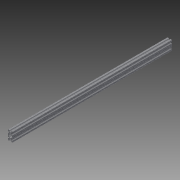
# Autodesk Inventor part: 1530-50_5
Saved by Autodesk Inventor 2013 (Build 170138000, 138)
## iProperties
Category: PARTsolutions
Company: 8020
Created: 2013-09-15
Part Number: 1530-50_5
Catalog Web Link: www.cadenas.de
Description: 1530-T-Slotted Profile - 15 Series
Vendor: 8020
Document SubType Name: Modeling
Designer: PARTuser1
Manufacturer: 8020
Density: 1 g/cm^3
Material: Generic
Mass: 1722.42 g
Surface Area: 7668.33 cm^2
Volume: 1722.42 cm^3
PSOL_IDENT_0: {$CADENAS_DATA\23d-libs\8020\inch\profiles\15_series\1530.prj},149 {VTYP=3D},{NB=1530-97},{LINA=1530
PSOL_IDENT_1: -97},{NN=1530},{DATE=22.08.2012},{GEOMDATE=16.08.2012 10:03:00},{VERSION=},{LINEID=10},{LINESUBID=-1
PSOL_IDENT_2: },{WBVAR=LS,L}  {NB=1530-97},{LINA=1530-97},{KT=DUMMY},{PN=1530-97},{SERIES=1530},{MAT=6105-T5 Alumi
PSOL_IDENT_3: num},{FIN=Clear Anodize},{LS=},{L=97.000},{LALG=97,145,242},{W=2.4209},{MIX=1.8042},{MIY=.4824},{EA=
PSOL_IDENT_4: 2.0798}
CNS_NT: T-Slotted Profile - 15 Series
CNS_NB: 1530-97
CNS_NBSYN: $PN.$LS.
CNS_LINA: 1530-97
CNS_PN: 1530-97
CNS_SERIES: 1530
CNS_MAT: 6105-T5 Aluminum
CNS_FIN: Clear Anodize
CNS_LS: Stock Length
CNS_L: 97.000
CNS_LALG: 97,145,242
CNS_W: 2.4209
CNS_MIX: 1.8042
CNS_MIY: .4824
CNS_EA: 2.0798
SUPPLIER: 8020
ARTICLENO: 1530-97
BOMINFO: 1530-97
CREATOR: CADENAS GmbH
Title: 1530-97
Author: Cadenas PARTsolutions
Comments: T-Slotted Profile - 15 Series
Autodesk Inventor part; units mm, degrees
sketch "Sketch_1" plane through (0, 0, 0) normal (0, 0, 1) x (1, 0, 0)
  arc A0 (-19.05, -15.8496) -> (-19.05, -14.3256) centre (-19.05, -15.0876) ccw
  line L0 (-19.05, -15.8496) -> (-19.05, -15.875)
  arc A1 (-19.05, -15.875) -> (-15.875, -19.05) centre (-15.875, -15.875) ccw
  line L1 (-15.875, -19.05) -> (-15.8496, -19.05)
  arc A2 (-14.3256, -19.05) -> (-15.8496, -19.05) centre (-15.0876, -19.05) ccw
  line L2 (-14.3256, -19.05) -> (-9.4996, -19.05)
  arc A3 (-7.9756, -19.05) -> (-9.4996, -19.05) centre (-8.7376, -19.05) ccw
  line L3 (-7.9756, -19.05) -> (-5.6388, -19.05)
  arc A4 (-5.6388, -19.05) -> (-4.064, -17.4752) centre (-5.6388, -17.4752) ccw
  line L4 (-4.064, -17.4752) -> (-4.064, -16.5608)
  arc A5 (-4.064, -16.5608) -> (-5.6388, -14.986) centre (-5.6388, -16.5608) ccw
  line L5 (-5.6388, -14.986) -> (-9.398, -14.986)
  arc A6 (-10.287, -14.097) -> (-9.398, -14.986) centre (-9.398, -14.097) ccw
  line L6 (-10.287, -14.097) -> (-10.287, -13.5289)
  arc A7 (-10.0266, -12.9003) -> (-10.287, -13.5289) centre (-9.398, -13.5289) ccw
  line L7 (-10.0266, -12.9003) -> (-5.2739, -8.1476)
  arc A8 (-1.9153, -6.7564) -> (-5.2739, -8.1476) centre (-1.9153, -11.5062) ccw
  line L8 (-1.9153, -6.7564) -> (1.9153, -6.7564)
  arc A9 (5.2739, -8.1476) -> (1.9153, -6.7564) centre (1.9153, -11.5062) ccw
  line L9 (5.2739, -8.1476) -> (10.0266, -12.9003)
  arc A10 (10.287, -13.5289) -> (10.0266, -12.9003) centre (9.398, -13.5289) ccw
  line L10 (10.287, -13.5289) -> (10.287, -14.097)
  arc A11 (9.398, -14.986) -> (10.287, -14.097) centre (9.398, -14.097) ccw
  line L11 (9.398, -14.986) -> (5.6388, -14.986)
  arc A12 (5.6388, -14.986) -> (4.064, -16.5608) centre (5.6388, -16.5608) ccw
  line L12 (4.064, -16.5608) -> (4.064, -17.4752)
  arc A13 (4.064, -17.4752) -> (5.6388, -19.05) centre (5.6388, -17.4752) ccw
  line L13 (5.6388, -19.05) -> (7.9756, -19.05)
  arc A14 (9.4996, -19.05) -> (7.9756, -19.05) centre (8.7376, -19.05) ccw
  line L14 (9.4996, -19.05) -> (12.7, -19.05)
  line L15 (12.7, -19.05) -> (14.3256, -19.05)
  arc A15 (15.8496, -19.05) -> (14.3256, -19.05) centre (15.0876, -19.05) ccw
  line L16 (15.8496, -19.05) -> (15.875, -19.05)
  arc A16 (15.875, -19.05) -> (19.05, -15.875) centre (15.875, -15.875) ccw
  line L17 (19.05, -15.875) -> (19.05, -15.8496)
  arc A17 (19.05, -14.3256) -> (19.05, -15.8496) centre (19.05, -15.0876) ccw
  line L18 (19.05, -14.3256) -> (19.05, -12.7)
  line L19 (19.05, -12.7) -> (19.05, -9.4996)
  arc A18 (19.05, -7.9756) -> (19.05, -9.4996) centre (19.05, -8.7376) ccw
  line L20 (19.05, -7.9756) -> (19.05, -5.6388)
  arc A19 (19.05, -5.6388) -> (17.4752, -4.064) centre (17.4752, -5.6388) ccw
  line L21 (17.4752, -4.064) -> (16.5608, -4.064)
  arc A20 (16.5608, -4.064) -> (14.986, -5.6388) centre (16.5608, -5.6388) ccw
  line L22 (14.986, -5.6388) -> (14.986, -9.398)
  arc A21 (14.097, -10.287) -> (14.986, -9.398) centre (14.097, -9.398) ccw
  line L23 (14.097, -10.287) -> (13.5289, -10.287)
  arc A22 (12.9003, -10.0266) -> (13.5289, -10.287) centre (13.5289, -9.398) ccw
  line L24 (12.9003, -10.0266) -> (8.1476, -5.2739)
  arc A23 (6.7564, -1.9153) -> (8.1476, -5.2739) centre (11.5062, -1.9153) ccw
  line L25 (6.7564, -1.9153) -> (6.7564, 1.9153)
  arc A24 (8.1476, 5.2739) -> (6.7564, 1.9153) centre (11.5062, 1.9153) ccw
  line L26 (8.1476, 5.2739) -> (12.9003, 10.0266)
  arc A25 (13.5289, 10.287) -> (12.9003, 10.0266) centre (13.5289, 9.398) ccw
  line L27 (13.5289, 10.287) -> (14.097, 10.287)
  arc A26 (14.986, 9.398) -> (14.097, 10.287) centre (14.097, 9.398) ccw
  line L28 (14.986, 9.398) -> (14.986, 5.6388)
  arc A27 (14.986, 5.6388) -> (16.5608, 4.064) centre (16.5608, 5.6388) ccw
  line L29 (16.5608, 4.064) -> (17.4752, 4.064)
  arc A28 (17.4752, 4.064) -> (19.05, 5.6388) centre (17.4752, 5.6388) ccw
  line L30 (19.05, 5.6388) -> (19.05, 7.9756)
  arc A29 (19.05, 9.4996) -> (19.05, 7.9756) centre (19.05, 8.7376) ccw
  line L31 (19.05, 9.4996) -> (19.05, 12.7)
  line L32 (19.05, 12.7) -> (19.05, 14.3256)
  arc A30 (19.05, 15.8496) -> (19.05, 14.3256) centre (19.05, 15.0876) ccw
  line L33 (19.05, 15.8496) -> (19.05, 22.2504)
  arc A31 (19.05, 23.7744) -> (19.05, 22.2504) centre (19.05, 23.0124) ccw
  line L34 (19.05, 23.7744) -> (19.05, 25.4)
  line L35 (19.05, 25.4) -> (19.05, 28.6004)
  arc A32 (19.05, 30.1244) -> (19.05, 28.6004) centre (19.05, 29.3624) ccw
  line L36 (19.05, 30.1244) -> (19.05, 32.4612)
  arc A33 (19.05, 32.4612) -> (17.4752, 34.036) centre (17.4752, 32.4612) ccw
  line L37 (17.4752, 34.036) -> (16.5608, 34.036)
  arc A34 (16.5608, 34.036) -> (14.986, 32.4612) centre (16.5608, 32.4612) ccw
  line L38 (14.986, 32.4612) -> (14.986, 28.702)
  arc A35 (14.097, 27.813) -> (14.986, 28.702) centre (14.097, 28.702) ccw
  line L39 (14.097, 27.813) -> (13.5289, 27.813)
  arc A36 (12.9003, 28.0734) -> (13.5289, 27.813) centre (13.5289, 28.702) ccw
  line L40 (12.9003, 28.0734) -> (8.1476, 32.8261)
  arc A37 (6.7564, 36.1847) -> (8.1476, 32.8261) centre (11.5062, 36.1847) ccw
  line L41 (6.7564, 36.1847) -> (6.7564, 40.0153)
  arc A38 (8.1476, 43.3739) -> (6.7564, 40.0153) centre (11.5062, 40.0153) ccw
  line L42 (8.1476, 43.3739) -> (12.9003, 48.1266)
  arc A39 (13.5289, 48.387) -> (12.9003, 48.1266) centre (13.5289, 47.498) ccw
  line L43 (13.5289, 48.387) -> (14.097, 48.387)
  arc A40 (14.986, 47.498) -> (14.097, 48.387) centre (14.097, 47.498) ccw
  line L44 (14.986, 47.498) -> (14.986, 43.7388)
  arc A41 (14.986, 43.7388) -> (16.5608, 42.164) centre (16.5608, 43.7388) ccw
  line L45 (16.5608, 42.164) -> (17.4752, 42.164)
  arc A42 (17.4752, 42.164) -> (19.05, 43.7388) centre (17.4752, 43.7388) ccw
  line L46 (19.05, 43.7388) -> (19.05, 46.0756)
  arc A43 (19.05, 47.5996) -> (19.05, 46.0756) centre (19.05, 46.8376) ccw
  line L47 (19.05, 47.5996) -> (19.05, 50.8)
  line L48 (19.05, 50.8) -> (19.05, 52.4256)
  arc A44 (19.05, 53.9496) -> (19.05, 52.4256) centre (19.05, 53.1876) ccw
  line L49 (19.05, 53.9496) -> (19.05, 53.975)
  arc A45 (19.05, 53.975) -> (15.875, 57.15) centre (15.875, 53.975) ccw
  line L50 (15.875, 57.15) -> (15.8496, 57.15)
  arc A46 (14.3256, 57.15) -> (15.8496, 57.15) centre (15.0876, 57.15) ccw
  line L51 (14.3256, 57.15) -> (12.7, 57.15)
  line L52 (12.7, 57.15) -> (9.4996, 57.15)
  arc A47 (7.9756, 57.15) -> (9.4996, 57.15) centre (8.7376, 57.15) ccw
  line L53 (7.9756, 57.15) -> (5.6388, 57.15)
  arc A48 (5.6388, 57.15) -> (4.064, 55.5752) centre (5.6388, 55.5752) ccw
  line L54 (4.064, 55.5752) -> (4.064, 54.6608)
  arc A49 (4.064, 54.6608) -> (5.6388, 53.086) centre (5.6388, 54.6608) ccw
  line L55 (5.6388, 53.086) -> (9.398, 53.086)
  arc A50 (10.287, 52.197) -> (9.398, 53.086) centre (9.398, 52.197) ccw
  line L56 (10.287, 52.197) -> (10.287, 51.6289)
  arc A51 (10.0266, 51.0003) -> (10.287, 51.6289) centre (9.398, 51.6289) ccw
  line L57 (10.0266, 51.0003) -> (5.2739, 46.2476)
  arc A52 (1.9153, 44.8564) -> (5.2739, 46.2476) centre (1.9153, 49.6062) ccw
  line L58 (1.9153, 44.8564) -> (-1.9153, 44.8564)
  arc A53 (-5.2739, 46.2476) -> (-1.9153, 44.8564) centre (-1.9153, 49.6062) ccw
  line L59 (-5.2739, 46.2476) -> (-10.0266, 51.0003)
  arc A54 (-10.287, 51.6289) -> (-10.0266, 51.0003) centre (-9.398, 51.6289) ccw
  line L60 (-10.287, 51.6289) -> (-10.287, 52.197)
  arc A55 (-9.398, 53.086) -> (-10.287, 52.197) centre (-9.398, 52.197) ccw
  line L61 (-9.398, 53.086) -> (-5.6388, 53.086)
  arc A56 (-5.6388, 53.086) -> (-4.064, 54.6608) centre (-5.6388, 54.6608) ccw
  line L62 (-4.064, 54.6608) -> (-4.064, 55.5752)
  arc A57 (-4.064, 55.5752) -> (-5.6388, 57.15) centre (-5.6388, 55.5752) ccw
  line L63 (-5.6388, 57.15) -> (-7.9756, 57.15)
  arc A58 (-9.4996, 57.15) -> (-7.9756, 57.15) centre (-8.7376, 57.15) ccw
  line L64 (-9.4996, 57.15) -> (-12.7, 57.15)
  line L65 (-12.7, 57.15) -> (-14.3256, 57.15)
  arc A59 (-15.8496, 57.15) -> (-14.3256, 57.15) centre (-15.0876, 57.15) ccw
  line L66 (-15.8496, 57.15) -> (-15.875, 57.15)
  arc A60 (-15.875, 57.15) -> (-19.05, 53.975) centre (-15.875, 53.975) ccw
  line L67 (-19.05, 53.975) -> (-19.05, 53.9496)
  arc A61 (-19.05, 52.4256) -> (-19.05, 53.9496) centre (-19.05, 53.1876) ccw
  line L68 (-19.05, 52.4256) -> (-19.05, 50.8)
  line L69 (-19.05, 50.8) -> (-19.05, 47.5996)
  arc A62 (-19.05, 46.0756) -> (-19.05, 47.5996) centre (-19.05, 46.8376) ccw
  line L70 (-19.05, 46.0756) -> (-19.05, 43.7388)
  arc A63 (-19.05, 43.7388) -> (-17.4752, 42.164) centre (-17.4752, 43.7388) ccw
  line L71 (-17.4752, 42.164) -> (-16.5608, 42.164)
  arc A64 (-16.5608, 42.164) -> (-14.986, 43.7388) centre (-16.5608, 43.7388) ccw
  line L72 (-14.986, 43.7388) -> (-14.986, 47.498)
  arc A65 (-14.097, 48.387) -> (-14.986, 47.498) centre (-14.097, 47.498) ccw
  line L73 (-14.097, 48.387) -> (-13.5289, 48.387)
  arc A66 (-12.9003, 48.1266) -> (-13.5289, 48.387) centre (-13.5289, 47.498) ccw
  line L74 (-12.9003, 48.1266) -> (-8.1476, 43.3739)
  arc A67 (-6.7564, 40.0153) -> (-8.1476, 43.3739) centre (-11.5062, 40.0153) ccw
  line L75 (-6.7564, 40.0153) -> (-6.7564, 36.1847)
  arc A68 (-8.1476, 32.8261) -> (-6.7564, 36.1847) centre (-11.5062, 36.1847) ccw
  line L76 (-8.1476, 32.8261) -> (-12.9003, 28.0734)
  arc A69 (-13.5289, 27.813) -> (-12.9003, 28.0734) centre (-13.5289, 28.702) ccw
  line L77 (-13.5289, 27.813) -> (-14.097, 27.813)
  arc A70 (-14.986, 28.702) -> (-14.097, 27.813) centre (-14.097, 28.702) ccw
  line L78 (-14.986, 28.702) -> (-14.986, 32.4612)
  arc A71 (-14.986, 32.4612) -> (-16.5608, 34.036) centre (-16.5608, 32.4612) ccw
  line L79 (-16.5608, 34.036) -> (-17.4752, 34.036)
  arc A72 (-17.4752, 34.036) -> (-19.05, 32.4612) centre (-17.4752, 32.4612) ccw
  line L80 (-19.05, 32.4612) -> (-19.05, 30.1244)
  arc A73 (-19.05, 28.6004) -> (-19.05, 30.1244) centre (-19.05, 29.3624) ccw
  line L81 (-19.05, 28.6004) -> (-19.05, 25.4)
  line L82 (-19.05, 25.4) -> (-19.05, 23.7744)
  arc A74 (-19.05, 22.2504) -> (-19.05, 23.7744) centre (-19.05, 23.0124) ccw
  line L83 (-19.05, 22.2504) -> (-19.05, 15.8496)
  arc A75 (-19.05, 14.3256) -> (-19.05, 15.8496) centre (-19.05, 15.0876) ccw
  line L84 (-19.05, 14.3256) -> (-19.05, 12.7)
  line L85 (-19.05, 12.7) -> (-19.05, 9.4996)
  arc A76 (-19.05, 7.9756) -> (-19.05, 9.4996) centre (-19.05, 8.7376) ccw
  line L86 (-19.05, 7.9756) -> (-19.05, 5.6388)
  arc A77 (-19.05, 5.6388) -> (-17.4752, 4.064) centre (-17.4752, 5.6388) ccw
  line L87 (-17.4752, 4.064) -> (-16.5608, 4.064)
  arc A78 (-16.5608, 4.064) -> (-14.986, 5.6388) centre (-16.5608, 5.6388) ccw
  line L88 (-14.986, 5.6388) -> (-14.986, 9.398)
  arc A79 (-14.097, 10.287) -> (-14.986, 9.398) centre (-14.097, 9.398) ccw
  line L89 (-14.097, 10.287) -> (-13.5289, 10.287)
  arc A80 (-12.9003, 10.0266) -> (-13.5289, 10.287) centre (-13.5289, 9.398) ccw
  line L90 (-12.9003, 10.0266) -> (-8.1476, 5.2739)
  arc A81 (-6.7564, 1.9153) -> (-8.1476, 5.2739) centre (-11.5062, 1.9153) ccw
  line L91 (-6.7564, 1.9153) -> (-6.7564, -1.9153)
  arc A82 (-8.1476, -5.2739) -> (-6.7564, -1.9153) centre (-11.5062, -1.9153) ccw
  line L92 (-8.1476, -5.2739) -> (-12.9003, -10.0266)
  arc A83 (-13.5289, -10.287) -> (-12.9003, -10.0266) centre (-13.5289, -9.398) ccw
  line L93 (-13.5289, -10.287) -> (-14.097, -10.287)
  arc A84 (-14.986, -9.398) -> (-14.097, -10.287) centre (-14.097, -9.398) ccw
  line L94 (-14.986, -9.398) -> (-14.986, -5.6388)
  arc A85 (-14.986, -5.6388) -> (-16.5608, -4.064) centre (-16.5608, -5.6388) ccw
  line L95 (-16.5608, -4.064) -> (-17.4752, -4.064)
  arc A86 (-17.4752, -4.064) -> (-19.05, -5.6388) centre (-17.4752, -5.6388) ccw
  line L96 (-19.05, -5.6388) -> (-19.05, -7.9756)
  arc A87 (-19.05, -9.4996) -> (-19.05, -7.9756) centre (-19.05, -8.7376) ccw
  line L97 (-19.05, -9.4996) -> (-19.05, -12.7)
  line L98 (-19.05, -12.7) -> (-19.05, -14.3256)
  circle A88 centre (0, 38.1) radius 3.3274
  circle A89 centre (0, 0) radius 3.3274
  arc A90 (-14.1109, 21.1155) -> (-14.1109, 16.9845) centre (-12.0454, 19.05) ccw
  line L99 (-14.1109, 16.9845) -> (-5.2739, 8.1476)
  arc A91 (-5.2739, 8.1476) -> (-1.9153, 6.7564) centre (-1.9153, 11.5062) ccw
  line L100 (-1.9153, 6.7564) -> (1.9153, 6.7564)
  arc A92 (1.9153, 6.7564) -> (5.2739, 8.1476) centre (1.9153, 11.5062) ccw
  line L101 (5.2739, 8.1476) -> (14.1109, 16.9845)
  arc A93 (14.1109, 16.9845) -> (14.1109, 21.1155) centre (12.0454, 19.05) ccw
  line L102 (14.1109, 21.1155) -> (5.2739, 29.9524)
  arc A94 (5.2739, 29.9524) -> (1.9153, 31.3436) centre (1.9153, 26.5938) ccw
  line L103 (1.9153, 31.3436) -> (-1.9153, 31.3436)
  arc A95 (-1.9153, 31.3436) -> (-5.2739, 29.9524) centre (-1.9153, 26.5938) ccw
  line L104 (-5.2739, 29.9524) -> (-14.1109, 21.1155)
  constraints: 210 end point, 188 point on circle, 96 centre point
extrude "Extrusion1" add sketch "Sketch_1" against normal blind 1282.7
ref_plane "b1_XY" through (0, -19.05, -1231.9) normal (0, 1, 0) x (1, 0, 0)
ref_plane "b1_YZ" through (0, -19.05, -1231.9) normal (1, 0, 0) x (0, 0, -1)
ref_plane "b1_ZX" through (0, -19.05, -1231.9) normal (0, 0, -1) x (0, 1, 0)
ref_plane "b2_XY" through (0, 57.15, -1231.9) normal (0, 1, 0) x (1, 0, 0)
ref_plane "b2_YZ" through (0, 57.15, -1231.9) normal (1, 0, 0) x (0, 0, -1)
ref_plane "b2_ZX" through (0, 57.15, -1231.9) normal (0, 0, -1) x (0, 1, 0)
ref_plane "profile1530_XY" through (0, 19.05, -1231.9) normal (0, 0, 1) x (1, 0, 0)
ref_plane "profile1530_YZ" through (0, 19.05, -1231.9) normal (1, 0, 0) x (0, 1, 0)
ref_plane "profile1530_ZX" through (0, 19.05, -1231.9) normal (0, 1, 0) x (0, 0, 1)
body "Solid1"
